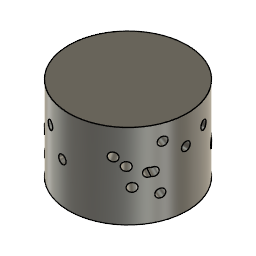
SPiDR_stencil_parametric (Autodesk Fusion 360 design; units mm, degrees)
part number: 2026-06-04-01-32-15-212
Autodesk Fusion 360 part; units mm, degrees
sketch "스케치1" plane through (0, 0, 0) normal (0, 0, 1) x (1, 0, 0)
  circle A0 centre (0, 0) radius 14
extrude "돌출1" add sketch "스케치1" along normal blind 20
sketch "스케치2" plane through (0, 0, 0) normal (0, 0, 1) x (1, 0, 0)
  circle A0 centre (0, 0) radius 8.5
extrude "돌출2" cut sketch "스케치2" along normal blind 17
ref_plane "작업 평면1" through (0, 0, 12.125) normal (-0.728969, -0.684547, 0) x (0, 0, 1)
sketch "스케치3" plane through (0, 0, 0) normal (-0.728969, -0.684547, 0) x (0, 0, 1)
  circle A0 centre (9.5, 0) radius 1
extrude "돌출3" cut sketch "스케치3" along normal blind 15
ref_plane "작업 평면2" through (0, 0, 12.125) normal (-0.928486, -0.371368, 0) x (0, 0, 1)
sketch "스케치4" plane through (0, 0, 0) normal (-0.928486, -0.371368, 0) x (0, 0, 1)
  circle A0 centre (2.5, 0) radius 1
extrude "돌출4" cut sketch "스케치4" along normal blind 15
ref_plane "작업 평면3" through (0, 0, 12.125) normal (0.999816, -0.019197, 0) x (0, 0, 1)
sketch "스케치5" plane through (0, 0, 0) normal (0.999816, -0.019197, 0) x (0, 0, 1)
  circle A0 centre (13.4, 0) radius 1
extrude "돌출5" cut sketch "스케치5" along normal blind 15
ref_plane "작업 평면4" through (0, 0, 12.125) normal (-0.795473, -0.605988, 0) x (0, 0, 1)
sketch "스케치6" plane through (0, 0, 0) normal (-0.795473, -0.605988, 0) x (0, 0, 1)
  circle A0 centre (3.7, 0) radius 1
extrude "돌출6" cut sketch "스케치6" along normal blind 15
ref_plane "작업 평면5" through (0, 0, 12.125) normal (0.692143, -0.72176, 0) x (0, 0, 1)
sketch "스케치7" plane through (0, 0, 0) normal (0.692143, -0.72176, 0) x (0, 0, 1)
  circle A0 centre (12, 0) radius 1
extrude "돌출7" cut sketch "스케치7" along normal blind 15
ref_plane "작업 평면6" through (0, 0, 12.125) normal (-0.118404, -0.992966, 0) x (0, 0, 1)
sketch "스케치8" plane through (0, 0, 0) normal (-0.118404, -0.992966, 0) x (0, 0, 1)
  circle A0 centre (9.7, 0) radius 1
extrude "돌출8" cut sketch "스케치8" along normal blind 15
ref_plane "작업 평면7" through (0, 0, 12.125) normal (0.936672, -0.350207, 0) x (0, 0, 1)
sketch "스케치9" plane through (0, 0, 0) normal (0.936672, -0.350207, 0) x (0, 0, 1)
  circle A0 centre (16.3, 0) radius 1
extrude "돌출9" cut sketch "스케치9" along normal blind 15
ref_plane "작업 평면8" through (0, 0, 12.125) normal (-0.395546, -0.918446, 0) x (0, 0, 1)
sketch "스케치10" plane through (0, 0, 0) normal (-0.395546, -0.918446, 0) x (0, 0, 1)
  circle A0 centre (14.3, 0) radius 1
extrude "돌출10" cut sketch "스케치10" along normal blind 15
ref_plane "작업 평면9" through (0, 0, 12.125) normal (-0.999048, 0.043619, 0) x (0, 0, 1)
sketch "스케치11" plane through (0, 0, 0) normal (-0.999048, 0.043619, 0) x (0, 0, 1)
  circle A0 centre (14, 0) radius 1
extrude "돌출11" cut sketch "스케치11" along normal blind 15
ref_plane "작업 평면10" through (0, 0, 12.125) normal (-0.243615, 0.969872, 0) x (0, 0, 1)
sketch "스케치12" plane through (0, 0, 0) normal (-0.243615, 0.969872, 0) x (0, 0, 1)
  circle A0 centre (10.7, 0) radius 1
extrude "돌출12" cut sketch "스케치12" along normal blind 15
ref_plane "작업 평면11" through (0, 0, 12.125) normal (0.889416, -0.457098, 0) x (0, 0, 1)
sketch "스케치13" plane through (0, 0, 0) normal (0.889416, -0.457098, 0) x (0, 0, 1)
  circle A0 centre (10.5, 0) radius 1
extrude "돌출13" cut sketch "스케치13" along normal blind 15
ref_plane "작업 평면12" through (0, 0, 12.125) normal (0.941471, 0.337095, 0) x (0, 0, 1)
sketch "스케치14" plane through (0, 0, 0) normal (0.941471, 0.337095, 0) x (0, 0, 1)
  circle A0 centre (14.9, 0) radius 1
extrude "돌출14" cut sketch "스케치14" along normal blind 15
ref_plane "작업 평면13" through (0, 0, 12.125) normal (0.56928, -0.822144, 0) x (0, 0, 1)
sketch "스케치15" plane through (0, 0, 0) normal (0.56928, -0.822144, 0) x (0, 0, 1)
  circle A0 centre (13.8, 0) radius 1
extrude "돌출15" cut sketch "스케치15" along normal blind 15
ref_plane "작업 평면14" through (0, 0, 12.125) normal (0.740805, -0.671721, 0) x (0, 0, 1)
sketch "스케치16" plane through (0, 0, 0) normal (0.740805, -0.671721, 0) x (0, 0, 1)
  circle A0 centre (7.7, 0) radius 1
extrude "돌출16" cut sketch "스케치16" along normal blind 15
ref_plane "작업 평면15" through (0, 0, 12.125) normal (-0.562083, 0.827081, 0) x (0, 0, 1)
sketch "스케치17" plane through (0, 0, 0) normal (-0.562083, 0.827081, 0) x (0, 0, 1)
  circle A0 centre (7.5, 0) radius 1
extrude "돌출17" cut sketch "스케치17" along normal blind 15
ref_plane "작업 평면16" through (0, 0, 12.125) normal (0.618408, 0.785857, 0) x (0, 0, 1)
sketch "스케치18" plane through (0, 0, 0) normal (0.618408, 0.785857, 0) x (0, 0, 1)
  circle A0 centre (6.8, 0) radius 1
extrude "돌출18" cut sketch "스케치18" along normal blind 15
ref_plane "작업 평면17" through (0, 0, 12.125) normal (0.858065, -0.513541, 0) x (0, 0, 1)
sketch "스케치19" plane through (0, 0, 0) normal (0.858065, -0.513541, 0) x (0, 0, 1)
  circle A0 centre (10.5, 0) radius 1
extrude "돌출19" cut sketch "스케치19" along normal blind 15
ref_plane "작업 평면18" through (0, 0, 12.125) normal (0.925871, -0.377841, 0) x (0, 0, 1)
sketch "스케치20" plane through (0, 0, 0) normal (0.925871, -0.377841, 0) x (0, 0, 1)
  circle A0 centre (5.8, 0) radius 1
extrude "돌출20" cut sketch "스케치20" along normal blind 15
ref_plane "작업 평면19" through (0, 0, 12.125) normal (-0.322266, 0.946649, 0) x (0, 0, 1)
sketch "스케치21" plane through (0, 0, 0) normal (-0.322266, 0.946649, 0) x (0, 0, 1)
  circle A0 centre (12.9, 0) radius 1
extrude "돌출21" cut sketch "스케치21" along normal blind 15
ref_plane "작업 평면20" through (0, 0, 12.125) normal (0.763796, 0.645458, 0) x (0, 0, 1)
sketch "스케치22" plane through (0, 0, 0) normal (0.763796, 0.645458, 0) x (0, 0, 1)
  circle A0 centre (7.7, 0) radius 1
extrude "돌출22" cut sketch "스케치22" along normal blind 15
named bodies: "SPiDR_Stencil"
